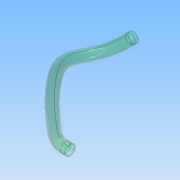
# Autodesk Inventor part: Top_Lower Pipe 3
Saved by Autodesk Inventor 2018.1 (Build 221171000, 171)
## iProperties
Created: 2019-03-21
Part Number: Top_Lower Pipe 3
Material: PMMA Plastic
Document SubType Name: Modeling
Designer: James
Density: 1.188 g/cm^3
Appearance: Clear - Green 1
Author: James
Autodesk Inventor part; units mm, degrees
ref_plane "YZ Plane" through (0, 0, 0) normal (1, 0, 0) x (0, 1, 0)
ref_plane "XZ Plane" through (0, 0, 0) normal (0, 1, 0) x (-1, 0, 0)
ref_plane "XY Plane" through (0, 0, 0) normal (0, 0, 1) x (1, 0, 0)
sketch "Sketch2" plane through (0, 0, 0) normal (0, 1, 0) x (-1, 0, 0)
  circle A0 centre (0, 0) radius 23
  circle A1 centre (0, 0) radius 20
  dimension "d1" = 46
  dimension "d2" = 40
  constraints: 2 centre point, 2 coincident
  measures "d1" diameter of A0
  measures "d2" diameter of A1
sketch3d "3D Sketch1"
  spline S0 degree 4 poles (0, 0, 0) (0, -180, 0) (-165, -180, 0) (-165, -180, -320) (-145, -180, -320) (-145, -180, -368) (-101, -180, -368) knots 1 1 1 1 1 2 3 4 4 4 4 4
  dimension "d33" = 180
  dimension "d34" = 165
  dimension "d35" = 320
  dimension "d37" = 48
  dimension "d38" = 44
  dimension "d39" = 20
sweep "Sweep1" add profiles "Sketch2" path "3D Sketch1"
sketch "Sketch3" plane through (0, 0, 0) normal (0, 1, 0) x (1, 0, 0)
  spline S0 degree 6 poles (-20, 0) (-20, 33.2309) (21.091, 38.0022) (54.9823, 0) (21.091, -38.0022) (-20, -33.2309) (-20, 0) knots 0 0 0 0 0 0 0 1 1 1 1 1 1 1 weights 1.669078 1.03673 1.038347 0.853534 1.038347 1.03673 1.669078 projected
  circle A0 centre (0, 0) radius 23 projected
  point P0 (-23, 0)
  constraints: 1 horizontal alignment, 1 other
extrude "Extrusion1" add sketch "Sketch3" along normal blind 12
sketch "Sketch4" plane through (0, 0, 0) normal (0, 0, 1) x (1, 0, 0)
  line L0 (23, 12) -> (-23, 12) projected
  point P0 (0, 0)
  point P1 (0, 5)
  point P2 (0, 12)
  dimension "d11" = 7
  constraints: 1 midpoint, 1 vertical alignment
  measures "d11" distance from line of L0 point (0, 5)
hole "Hole1" at (0, 5, 0) direction (0, 0, -1) diameter 4.5 end through all
sketch "Sketch5" plane through (-101, -180, -368) normal (1, 0, 0) x (0, 0, -1)
  spline S0 degree 6 poles (9.2914, 17.7107) (-20.1357, 33.1488) (-43.4506, -1.022) (-25.5432, -48.6888) (23.8541, -36.3316) (38.7185, 2.2726) (9.2914, 17.7107) knots 0 0 0 0 0 0 0 1 1 1 1 1 1 1 weights 1.669078 1.03673 1.038347 0.853534 1.038347 1.03673 1.669078 projected
  circle A0 centre (0, 0) radius 23 projected
  point P0 (-368, 180)
  point P1 (10.3268, 20.5513)
  constraints: 2 other
extrude "Extrusion2" add sketch "Sketch5" along normal blind 20 contours S0 picked at (-0.7718, -21.8434)
body "Solid1"
